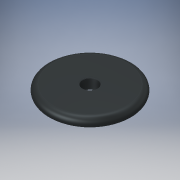
# Autodesk Inventor part: 5lb_weight
Saved by Autodesk Inventor 2019 (Build 230136000, 136)
## iProperties
Created: 2019-04-21
Part Number: 5lb_weight
Material: Iron, Cast
Document SubType Name: Modeling
Designer: Wilson Lab
Density: 7.15 g/cm^3
Appearance: Iron Gray
Mass: 2352.57 g
Surface Area: 433.03 cm^2
Volume: 329.03 cm^3
Author: Wilson Lab
Autodesk Inventor part; units mm, degrees
ref_plane "YZ Plane" through (0, 0, 0) normal (1, 0, 0) x (0, 1, 0)
ref_plane "XZ Plane" through (0, 0, 0) normal (0, 1, 0) x (-1, 0, 0)
ref_plane "XY Plane" through (0, 0, 0) normal (0, 0, 1) x (1, 0, 0)
sketch "Sketch1" plane through (0, 0, 0) normal (0, 1, 0) x (-1, 0, 0)
  circle A0 centre (0, 0) radius 77.47
  circle A1 centre (0, 0) radius 13.97
  dimension "d0" = 154.94
  dimension "d1" = 27.94
  constraints: 2 centre point, 2 coincident
  measures "d0" diameter of A0
  measures "d1" diameter of A1
extrude "Extrusion1" add sketch "Sketch1" along normal blind 19.05
fillet "Fillet1" radius 9.525 2 edges at (77.47, 19.05, 0) (77.47, 0, 0)
chamfer "Chamfer1" distance 0.635 angle 45 2 edges at (13.97, 19.05, 0) (13.97, 0, 0)
body "Solid1"
